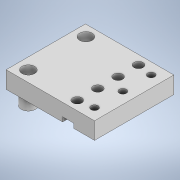
# Autodesk Inventor part: CameraAdapter_part1
Saved by Autodesk Inventor 2020.1 (Build 241239000, 239)
## iProperties
Created: 2019-09-03
Part Number: CameraAdapter_part1
Material: Generic
Document SubType Name: Modeling
Designer: Julian
Density: 1 g/cm^3
Appearance: Default
Author: Julian
Autodesk Inventor part; units mm, degrees
ref_plane "YZ Plane" through (0, 0, 0) normal (1, 0, 0) x (0, 1, 0)
ref_plane "XZ Plane" through (0, 0, 0) normal (0, 1, 0) x (-1, 0, 0)
ref_plane "XY Plane" through (0, 0, 0) normal (0, 0, 1) x (1, 0, 0)
sketch "Sketch1" plane through (0, 0, 0) normal (0, 1, 0) x (-1, 0, 0)
  line L0 (0, 0) -> (78, 0)
  line L1 (78, 0) -> (78, -70)
  line L2 (78, -70) -> (0, -70)
  line L3 (0, -70) -> (0, 0)
  line L4 (0, 0) -> (10, 0)
  line L5 (10, 0) -> (10, -70)
  line L6 (10, -70) -> (0, -70)
  line L7 (0, -70) -> (0, 0)
  line L8 (10, 0) -> (10, -10)
  line L9 (10, -10) -> (10, -34.9935)
  line L10 (10, -34.9935) -> (10, -59.987)
  line L11 (78, -70) -> (68, -70)
  line L12 (68, -70) -> (68, 0)
  line L13 (68, 0) -> (78, 0)
  line L14 (78, 0) -> (78, -70)
  line L15 (68, -70) -> (68, -60.4)
  line L16 (68, -60.4) -> (68, -9.6)
  circle A0 centre (68, -60.4) radius 6.25
  circle A1 centre (68, -9.6) radius 6.25
  line L17 (0, 0) -> (18.2, 0)
  line L18 (18.2, 0) -> (18.2, -70)
  line L19 (18.2, -70) -> (0, -70)
  line L20 (0, -70) -> (0, 0)
  line L21 (18.2, -70) -> (28.2, -70)
  line L22 (28.2, -70) -> (28.2, 0)
  line L23 (28.2, 0) -> (18.2, 0)
  line L24 (18.2, 0) -> (18.2, -70)
  dimension "d0" = 78
  dimension "d1" = 70
  dimension "d2" = 10
  dimension "d3" = 10
  dimension "d4" = 24.9935
  dimension "d5" = 24.9935
  dimension "d27" = 10
  dimension "d28" = 9.6
  dimension "d29" = 50.8
  dimension "d30" = 12.5
  dimension "d31" = 12.5
  dimension "d49" = 18.2
  dimension "d50" = 10
  constraints: 50 end point, 10 parallel, 9 point on line, 5 horizontal, 5 perpendicular, 2 centre point, 2 coincident
  measures "d0" distance of L1.end L2.end
  measures "d1" distance of L0.end L1.end
  measures "d2" distance of L5.end L6.end
  measures "d3" distance of L4.end L8.end
  measures "d4" distance of L8.end L9.end
  measures "d5" distance of L9.end L10.end
  measures "d27" distance of L12.end L13.end
  measures "d28" distance of L11.end L15.end
  measures "d29" distance of L15.end L16.end
  measures "d30" diameter of A0
  measures "d31" diameter of A1
  measures "d49" distance of L18.end L19.end
  measures "d50" distance of L23.end L22.end
extrude "Extrusion1" add sketch "Sketch1" along normal blind 15
sketch "Sketch2" plane through (0, 15, 0) normal (0, 1, 0) x (1, 0, 0)
  line L0 (-78, 70) -> (-78, 0) projected
  line L1 (-78, 0) -> (0, 0) projected
  line L2 (-78, 70) -> (-68, 70)
  line L3 (-68, 70) -> (-68, 0)
  line L4 (-68, 0) -> (-78, 0)
  line L5 (-78, 0) -> (-78, 70)
  line L6 (-68, 70) -> (-68, 60.4)
  line L7 (-68, 60.4) -> (-68, 9.6)
  line L8 (0, 70) -> (-78, 70) projected
  line L9 (-68, 0) -> (-28.2, 0)
  line L10 (-28.2, 0) -> (-28.2, 70)
  line L11 (-28.2, 70) -> (-68, 70)
  line L12 (-68, 70) -> (-68, 0)
  line L13 (-28.2, 70) -> (-18.2, 70)
  line L14 (-18.2, 70) -> (-18.2, 0)
  line L15 (-18.2, 0) -> (-28.2, 0)
  line L16 (-28.2, 0) -> (-28.2, 70)
  line L17 (-28.2, 0) -> (-23.2, 0)
  line L18 (-23.2, 0) -> (-23.2, 70)
  line L19 (-23.2, 70) -> (-28.2, 70)
  line L20 (-28.2, 70) -> (-28.2, 0)
  line L21 (-23.2, 0) -> (-23.2, 8)
  line L22 (-23.2, 8) -> (-23.2, 26)
  line L23 (-23.2, 26) -> (-23.2, 44)
  line L24 (-23.2, 44) -> (-23.2, 62)
  line L25 (-23.2, 62) -> (-23.2, 70)
  point P0 (-28.2, 0)
  dimension "d15" = 10
  dimension "d16" = 9.6
  dimension "d17" = 50.8
  dimension "d25" = 39.8
  dimension "d26" = 10
  dimension "d36" = 5
  dimension "d37" = 8
  dimension "d38" = 18
  dimension "d39" = 18
  dimension "d40" = 18
  dimension "d41" = 8
  constraints: 46 end point, 10 point on line, 8 parallel, 4 horizontal, 4 perpendicular, 1 midpoint
  measures "d15" distance of L3.end L4.end
  measures "d16" distance of L2.end L6.end
  measures "d17" distance of L6.end L7.end
  measures "d25" distance of L11.end L10.end
  measures "d26" distance of L14.end L15.end
  measures "d36" distance of L19.end L18.end
  measures "d37" distance of L17.end L21.end
  measures "d38" distance of L21.end L22.end
  measures "d39" distance of L22.end L23.end
  measures "d40" distance of L23.end L24.end
  measures "d41" distance of L24.end L25.end
extrude "Extrusion2" add sketch "Sketch1" against normal blind 12 contours A1 L12 | L12 A1 | A0 L12 | L12 A0
hole "Hole1" at (-10, 0, -10) at (-10, 0, -34.9935) at (-10, 0, -59.987) direction (0, 1, 0) diameter 6.2 end through all counterbore diameter 11 counterbore depth 8 clearance for "Socket Head Cap Screw" size "M6" standard "Ansi Metric M Profile"
hole "Hole2" at (-68, 15, -60.4) at (-68, 15, -9.6) direction (0, -1, 0) diameter 6.5 end through all counterbore diameter 11.113 counterbore depth 8 clearance for "Socket Head Cap Screw" size "1/4" standard "Ansi Unified Screw Threads"
hole "Hole3" at (-23.2, 15, -62) at (-23.2, 15, -44) at (-23.2, 15, -26) at (-23.2, 15, -8) direction (0, -1, 0) diameter 4.2 end through all counterbore diameter 8 counterbore depth 6 clearance for "Socket Head Cap Screw" size "M4" standard "Ansi Metric M Profile"
extrude "Extrusion4" cut sketch "Sketch1" along normal blind 4 contours L0 L22 L2 L18
body "Solid1"
